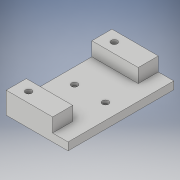
# Autodesk Inventor part: Backplate
Saved by Autodesk Inventor 2019 (Build 230136000, 136)
## iProperties
Created: 2021-06-02
Part Number: Backplate
Material: Generisch
Document SubType Name: Modeling
Designer: Bergi
Density: 1 g/cm^3
Appearance: Vorgabe
Author: Bergi
Autodesk Inventor part; units mm, degrees
ref_plane "YZ Plane" through (0, 0, 0) normal (1, 0, 0) x (0, 1, 0)
ref_plane "XZ Plane" through (0, 0, 0) normal (0, 1, 0) x (-1, 0, 0)
ref_plane "XY Plane" through (0, 0, 0) normal (0, 0, 1) x (1, 0, 0)
sketch "Skizze1" plane through (0, 0, 0) normal (0, 1, 0) x (-1, 0, 0)
  line L0 (-20, 34.2) -> (20, 34.2)
  line L1 (20, 34.2) -> (20, -34.2)
  line L2 (20, -34.2) -> (-20, -34.2)
  line L3 (-20, -34.2) -> (-20, 34.2)
  line L4 (-20, 34.2) -> (20, -34.2) construction
  line L5 (20, 34.2) -> (-20, -34.2) construction
  point P0 (0, 0)
  dimension "d0" = 40
  dimension "d1" = 68.4
  constraints: 12 end point, 2 midpoint, 2 parallel, 1 horizontal, 1 perpendicular
  measures "d0" distance of L1.end L2.end
  measures "d1" distance of L0.end L1.end
extrude "Extrusion1" add sketch "Skizze1" along normal blind 5
sketch "Skizze5" plane through (0, 0, 0) normal (0, -1, 0) x (1, 0, 0)
  line L0 (20, 34.2) -> (-20, 34.2) projected
  line L1 (-20, 34.2) -> (-20, -34.2) projected
  line L2 (-20, -34.2) -> (20, -34.2) projected
  line L3 (20, -34.2) -> (20, 34.2) projected
  line L4 (32.3204, 0) -> (-38.6965, 0) construction
  point P0 (0, 0)
  point P1 (-10, 0)
  point P2 (10, 0)
  dimension "d32" = 10
  dimension "d33" = 20
  constraints: 3 point on line, 2 end point, 1 horizontal
  measures "d32" distance from line of L1 point (-10, 0)
  measures "d33" distance of point (10, 0) point (-10, 0)
hole "Bohrung3" at (-10, 0, 0) at (10, 0, 0) direction (0, 1, 0) diameter 4 end through all counterbore diameter 8 counterbore depth 3
sketch "Skizze6" plane through (0, 5, 0) normal (0, 1, 0) x (1, 0, 0)
  circle A0 centre (-10, 0) radius 2 projected
  circle A1 centre (10, 0) radius 2 projected
  line L0 (-20, -34.2) -> (20, -34.2) projected
  line L1 (20, -34.2) -> (20, 34.2) projected
  line L2 (20, 34.2) -> (-20, 34.2) projected
  line L3 (-20, 34.2) -> (-20, -34.2) projected
  line L4 (-20, 34.2) -> (10, 34.2)
  line L5 (10, 34.2) -> (10, 21.2)
  line L6 (10, 21.2) -> (-20, 21.2)
  line L7 (-20, 21.2) -> (-20, 34.2)
  line L8 (-35, 0) -> (35, 0) projected
  line L9 (-20, -34.2) -> (10, -34.2)
  line L10 (10, -34.2) -> (10, -21.2)
  line L11 (10, -21.2) -> (-20, -21.2)
  line L12 (-20, -21.2) -> (-20, -34.2)
  point P0 (0, 0)
  dimension "d41" = 30
  dimension "d42" = 13
  constraints: 16 end point, 3 symmetric about line, 2 parallel, 1 horizontal, 1 perpendicular
  measures "d41" distance of L5.end L6.end
  measures "d42" distance of L4.end L5.end
extrude "Extrusion3" add sketch "Skizze6" along normal blind 9 contours L3 L2 L5 L6 | L11 L10 L0 L3
sketch "Skizze8" plane through (0, 0, 0) normal (0, -1, 0) x (1, 0, 0)
  line L0 (-20, 34.2) -> (10, 34.2) projected
  line L1 (10, 34.2) -> (10, 21.2) projected
  line L2 (10, 21.2) -> (-20, 21.2) projected
  line L3 (-20, 21.2) -> (-20, 34.2) projected
  line L4 (-20, -34.2) -> (-20, -21.2) projected
  line L5 (-20, -21.2) -> (10, -21.2) projected
  line L6 (10, -21.2) -> (10, -34.2) projected
  line L7 (10, -34.2) -> (-20, -34.2) projected
  line L8 (-20, 21.2) -> (-20, 34.2) projected
  line L9 (-20, 27.7) -> (10, 27.7)
  line L10 (-20, 34.2) -> (-20, -34.2) projected
  line L11 (10, -21.2) -> (10, -34.2) projected
  line L12 (10, -27.7) -> (-20, -27.7)
  point P0 (0, 0)
  point P1 (-12, 27.7)
  point P2 (-12, -27.7)
  dimension "d46" = 8
  dimension "d47" = 8
  constraints: 4 end point, 3 midpoint, 3 point on line, 1 perpendicular
  measures "d46" distance from line of L3 point (-12, 27.7)
  measures "d47" distance from line of L4 point (-12, -27.7)
hole "Bohrung4" at (-12, 0, 27.7) at (-12, 0, -27.7) direction (0, 1, 0) diameter 4 end through all counterbore diameter 7 counterbore depth 10
